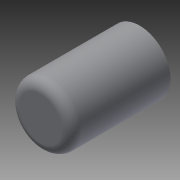
# Autodesk Inventor part: koncowka do laski - walec zaokraglony
Saved by Autodesk Inventor 2014 (Build 180170000, 170)
## iProperties
Created: 2017-01-10
Part Number: koncowka do laski - walec zaokraglony
Material: Ogólny
Document SubType Name: Modeling
Designer: hpdc7700
Density: 1 g/cm^3
Appearance: Domyślna
Author: hpdc7700
Autodesk Inventor part; units mm, degrees
ref_plane "YZ Plane" through (0, 0, 0) normal (1, 0, 0) x (0, 1, 0)
ref_plane "XZ Plane" through (0, 0, 0) normal (0, 1, 0) x (-1, 0, 0)
ref_plane "XY Plane" through (0, 0, 0) normal (0, 0, 1) x (1, 0, 0)
sketch "Szkic1" plane through (0, 0, 0) normal (0, 1, 0) x (-1, 0, 0)
  circle A0 centre (0, 0) radius 12.5
  dimension "d0" = 25
  constraints: 1 centre point, 1 coincident
  measures "d0" diameter of A0
extrude "Wyciągnięcie proste1" add sketch "Szkic1" along normal blind 40
fillet "Zaokrąglenie1" radius 4 1 edges at (12.5, 0, 0)
sketch "Szkic2" plane through (0, 40, 0) normal (0, 1, 0) x (1, 0, 0)
  circle A0 centre (0, 0) radius 12.5 projected
  circle A1 centre (0, 0) radius 8
  dimension "d4" = 16
  constraints: 1 centre point, 1 coincident
  measures "d4" diameter of A1
extrude "Wyciągnięcie proste2" cut sketch "Szkic2" against normal blind 20 contours A1
sketch "Szkic3" plane through (0, 20, 0) normal (0, 1, 0) x (1, 0, 0)
  circle A0 centre (0, 0) radius 8 projected
  circle A1 centre (0, 0) radius 4.5
  dimension "d7" = 9
  constraints: 1 centre point, 1 coincident
  measures "d7" diameter of A1
extrude "Wyciągnięcie proste3" cut sketch "Szkic3" against normal blind 6 contours A1
chamfer "Faza1" distance 0.5 angle 45 1 edges at (-4.5, 20, 0)
